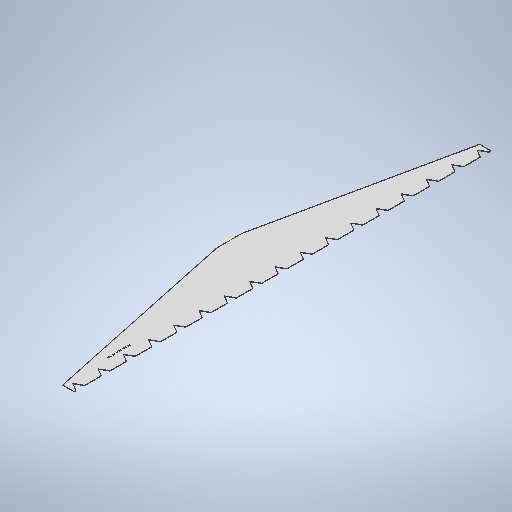
# Autodesk Inventor part: BSH 014 board cone_CPY
Saved by Autodesk Inventor 2025 (Build 290162010, 162A)
## iProperties
Created: 2024-07-23
Part Number: BSH 014 board cone_CPY
Material: 09g2s
Document SubType Name: Sheet Metal
Designer: admin
Stock Number: БШК 014 борт конус
Mass: 40581.4 g
Surface Area: 34651.2 cm^2
Volume: 5169.6 cm^3
Density: 7.85 g/cm^3
Flat Pattern Width: 42 cm
Flat Pattern Length: 330 cm
Flat Pattern Area: 13860 cm^2
Sheet Metal Rule: AISI304 3mm Die 32
Sheet Metal Width: 420,000 mm
Sheet Metal Length: 3300,000 mm
Sheet Metal Area: 1386000,000 mm^2
Appearance: Default
Author: admin
Autodesk Inventor part; units mm, degrees
ref_plane "YZ Plane" through (0, 0, 0) normal (1, 0, 0) x (0, 1, 0)
ref_plane "XZ Plane" through (0, 0, 0) normal (0, 1, 0) x (-1, 0, 0)
ref_plane "XY Plane" through (0, 0, 0) normal (0, 0, 1) x (1, 0, 0)
sketch "Sketch1" plane through (0, 0, 0) normal (0, 0, 1) x (1, 0, 0)
  line L0 (0, -1650) -> (420, -1650)
  line L1 (420, -1650) -> (420, 1650)
  line L2 (420, 1650) -> (0, 1650)
  line L3 (0, 1650) -> (0, -1650)
  line L4 (0, 0) -> (420, 0) construction
  line L5 (330, 1650) -> (0, 100)
  line L6 (0, -100) -> (330, -1650)
  dimension "d0" = 420
  dimension "d1" = 3300
  dimension "d41" = 200
  dimension "d42" = 90
  measures "d0" distance of L2.end L1.end
  measures "d1" distance of L1.end L0.end
  measures "d41" distance of L6.start L5.end
  measures "d42" distance of L5.start L1.end
extrude "Plate1" add sketch "Sketch1" along normal blind 3 contours L6 L3 L5 L2 L1 L0
sketch "Sketch5" plane through (0, 0, 0) normal (0, 0, -1) x (-1, 0, 0)
  line L0 (-330, -1650) -> (-420, -1650) construction
  line L1 (0, 100) -> (0, -100) projected
  line L2 (-420, 1650) -> (-330, 1650) construction
  line L3 (-420, -1650) -> (-420, 1650) projected
  line L4 (12.3081, -1975.0573) -> (-487.6919, -1975.0573)
  line L5 (-487.6919, -1975.0573) -> (-487.6919, -2425.2593)
  line L6 (-487.6919, -2425.2593) -> (12.3081, -1975.0573)
  line L7 (0, -100) -> (-330, -1650) projected
  line L8 (-330, 1650) -> (0, 100) projected
  line L9 (-420, 35) -> (-360, 0)
  line L10 (-360, 0) -> (-420, -35)
  point P0 (0, 0)
  point P1 (0, 0)
  point P2 (-420, 0)
  dimension "d26" = 500
  dimension "d27" = 48
  dimension "d28" = 672.8164
  dimension "d44" = 60
  dimension "d48" = 70
  constraints: 10 end point, 2 midpoint, 2 point on line, 1 equal length, 1 horizontal, 1 horizontal alignment, 1 perpendicular
  measures "d26" distance of L4.start L4.end
  measures "d27" angle of L6 L5
  measures "d28" distance of L5.end L4.start
  measures "d44" distance from line of L9.end L3
  measures "d48" distance of L9.start L10.end
extrude "Cut1" cut sketch "Sketch5" against normal blind 3 contours L3 L9 L10
sketch "Sketch8" plane through (0, 0, 0) normal (0, 0, -1) x (-1, 0, 0)
  point P0 (0, 0)
sketch "Sketch9" plane through (0, 0, 0) normal (0, 0, -1) x (-1, 0, 0)
  line L0 (-309.7791, -1281.5941) -> (-324.7791, -1281.5941) construction
  line L1 (-324.7791, -1281.5941) -> (-324.7791, -1081.5941) construction
  line L2 (-324.7791, -1081.5941) -> (-309.7791, -1081.5941) construction
  line L3 (-309.7791, -1081.5941) -> (-309.7791, -1281.5941) construction
  line L4 (-420, -1650) -> (-420, 1650) projected
  line L5 (-330, -1650) -> (-420, -1650) projected
  point P0 (0, 0)
  point P1 (0, -1650)
  dimension "d36" = 200
  dimension "d37" = 15
  constraints: 2 parallel, 2 other
  measures "d36" distance of L0.end L1.end
  measures "d37" distance between parallel lines of L1 L3
mark "Mark1"
pattern_linear "Rectangular Pattern2" count 18 spacing 200 along (0, 1, 0) of "Cut1" first direction both ways yes
equation "\"d31\" = Thickness"
equation "\"d2\" = Thickness"
equation "\"BendReliefWidth\" = Thickness"
equation "\"BendReliefDepth\" = 0.5 * Thickness"
equation "\"CornerReliefSize\" = 4 * Thickness"
equation "\"MinimumRemnant\" = 2 * Thickness"
equation "\"TransitionRadius\" = BendRadius"
equation "\"JacobiRadiusSize\" = BendRadius"
equation "\"GapSize\" = Thickness"
equation "\"Thickness\" = 3"
equation "\"BendRadius\" = 5"
body "Solid1"
